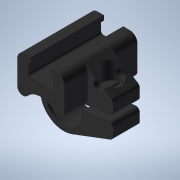
# Autodesk Inventor part: 175091 SMBR-8-8
Saved by Autodesk Inventor 2021 (Build 250183000, 183)
## iProperties
Created: 2026-04-13
Part Number: 175091 SMBR-8-8
Material: Generic
Catalog Web Link: www.3dfindit.com
Description: SMBR-Mounting kit
Vendor: FESTO
Document SubType Name: Modeling
Designer: psAdmin
Manufacturer: FESTO
Mass: 2.14298 g
Surface Area: 20.1199 cm^2
Volume: 2.14298 cm^3
Density: 1 g/cm^3
Appearance: PSOLRGB-176-176-176
Category: PARTsolutions
Company: FESTO
Title: 175091 SMBR-8-8
Author: Cadenas PARTsolutions
Comments: Mounting kit
PSOL_IDENT_0: {$CADENAS_DATA/23d-libs/festo/parts/s/smbr/smbr.prj},169 {VTYP=3D},{NB=175091 SMBR-8-8},{LINA=175091
PSOL_IDENT_1: SMBR-8-8},{NN=SMBR},{DATE=30.08.2023 07:56:14},{GEOMDATE=30.08.2023 07:02:41},{VERSION=},{LINEID=24
PSOL_IDENT_2: 0},{WBVAR=},{WBNUMERIC=}  {NB=175091 SMBR-8-8},{LINA=175091 SMBR-8-8},{KT=DUMMY},{TNR=175091},{TYP=S
PSOL_IDENT_3: MBR-8-8},{INFO=},{B1=18.900},{B2=12.300},{B3=7.000},{B4=0.000},{H1=17.500},{H2=0.000},{H3=0.000},{VE
PSOL_IDENT_4: RS=18.000},{FDTKDM=8},{EOLDATE=},{GTIN=4052568037772}
NB: 175091 SMBR-8-8
NN: SMBR
NT: Mounting kit
NBSYN: $TNR. $TYP.
LINA: 175091 SMBR-8-8
CATALOG: Festo
TNR: 175091
TYP: SMBR-8-8
B1: 18.9
B2: 12.3
B3: 7
B4: 0
H1: 17.5
H2: 0
H3: 0
GTIN: 4052568037772
SUPPLIER: FESTO
ARTICLENO: 175091 SMBR-8-8
BOMINFO: 175091 SMBR-8-8
CREATOR: CADENAS GmbH
Autodesk Inventor part; units mm, degrees
sketch "Skizze_1" plane through (0, 0, 0) normal (0, 0, 1) x (1, 0, 0)
  arc A0 (-6.1, 6.1) -> (2.1523, 0.3923) centre (0, 6.1) ccw
  line L0 (2.1523, 0.3923) -> (12.1528, 4.1634)
  arc A1 (12.1528, 4.1634) -> (12.8, 5.099) centre (11.8, 5.099) ccw
  line L1 (12.8, 5.099) -> (12.8, 7.1459)
  arc A2 (12.8, 7.1459) -> (11.6781, 8.1384) centre (11.8, 7.1459) ccw
  line L2 (11.6781, 8.1384) -> (5.5207, 7.3824)
  arc A3 (5.5207, 7.3824) -> (4.6439, 6.3385) centre (5.6426, 6.3898) ccw
  arc A4 (3.4991, 9.1625) -> (4.6439, 6.3385) centre (0, 6.1) ccw
  arc A5 (3.4991, 9.1625) -> (4.7232, 8.695) centre (4.5526, 10.0845) ccw
  line L3 (4.7232, 8.695) -> (11.9219, 9.5788)
  arc A6 (11.9219, 9.5788) -> (12.8, 10.5714) centre (11.8, 10.5714) ccw
  line L4 (12.8, 10.5714) -> (12.8, 12.6877)
  arc A7 (12.8, 12.6877) -> (12.3421, 13.528) centre (11.8, 12.6877) ccw
  line L5 (12.3421, 13.528) -> (10.513, 14.7078)
  arc A8 (10.513, 14.7078) -> (10.2108, 14.5895) centre (10.4045, 14.5398) ccw
  arc A9 (8.2178, 15.875) -> (10.2108, 14.5895) centre (9, 14.9) ccw
  arc A10 (8.2178, 15.875) -> (8.2011, 16.1991) centre (8.0927, 16.031) ccw
  line L6 (8.2011, 16.1991) -> (5.2841, 18.0807)
  arc A11 (5.2841, 18.0807) -> (4.2, 18.4) centre (4.2, 16.4) ccw
  line L7 (4.2, 18.4) -> (-4.1, 18.4)
  arc A12 (-4.1, 18.4) -> (-6.1, 16.4) centre (-4.1, 16.4) ccw
  line L8 (-6.1, 16.4) -> (-6.1, 6.1)
  constraints: 26 point on circle, 18 end point, 13 centre point
extrude "Extrusion1" add sketch "Skizze_1" along normal mid plane 7
sketch "Skizze_2" plane through (0, 0, 0) normal (0, 0, 1) x (1, 0, 0)
  line L0 (9, 0) -> (9, 18.4)
  line L1 (9, 18.4) -> (11.5, 18.4)
  line L2 (11.5, 18.4) -> (11.5, 11.1)
  line L3 (11.5, 11.1) -> (10.65, 11.1)
  line L4 (10.65, 11.1) -> (10.65, 6.6)
  line L5 (10.65, 6.6) -> (10.25, 6.6)
  line L6 (10.25, 6.6) -> (10.25, 5.1)
  line L7 (10.25, 5.1) -> (10.65, 5.1)
  line L8 (10.65, 5.1) -> (10.65, 0)
  line L9 (10.65, 0) -> (9, 0)
  line L10 (9, 0) -> (9, 18.4)
  constraints: 22 end point
revolve "Revolution1" cut sketch "Skizze_2" angle 360 about axis through (9, 0, 0) along (0, -1, 0)
sketch "Skizze_3" plane through (0, 0, 9.5) normal (0, 0, 1) x (1, 0, 0)
  arc A0 (-6.1, 10.182) -> (-3.478, 9.1864) centre (-4.6, 10.182) ccw
  arc A1 (3.5537, 9.099) -> (-3.478, 9.1864) centre (0, 6.1) ccw
  arc A2 (3.5537, 9.099) -> (6.2, 10.0664) centre (4.7, 10.0664) ccw
  line L0 (6.2, 10.0664) -> (6.2, 16.4)
  arc A3 (6.2, 16.4) -> (4.2, 18.4) centre (4.2, 16.4) ccw
  line L1 (4.2, 18.4) -> (-4.1, 18.4)
  arc A4 (-4.1, 18.4) -> (-6.1, 16.4) centre (-4.1, 16.4) ccw
  line L2 (-6.1, 16.4) -> (-6.1, 10.182)
  constraints: 10 point on circle, 6 end point, 5 centre point
extrude "Extrusion2" add sketch "Skizze_3" against normal blind 6
sketch "Skizze_4" plane through (0, 0, -9.5) normal (0, 0, 1) x (1, 0, 0)
  arc A0 (-6.1, 10.182) -> (-3.478, 9.1864) centre (-4.6, 10.182) ccw
  arc A1 (3.5537, 9.099) -> (-3.478, 9.1864) centre (0, 6.1) ccw
  arc A2 (3.5537, 9.099) -> (6.2, 10.0664) centre (4.7, 10.0664) ccw
  line L0 (6.2, 10.0664) -> (6.2, 16.4)
  arc A3 (6.2, 16.4) -> (4.2, 18.4) centre (4.2, 16.4) ccw
  line L1 (4.2, 18.4) -> (-4.1, 18.4)
  arc A4 (-4.1, 18.4) -> (-6.1, 16.4) centre (-4.1, 16.4) ccw
  line L2 (-6.1, 16.4) -> (-6.1, 10.182)
  constraints: 10 point on circle, 6 end point, 5 centre point
extrude "Extrusion3" add sketch "Skizze_4" along normal blind 6
sketch "Skizze_6" plane through (0, 0, 0) normal (0, 0, 1) x (1, 0, 0)
  line L0 (-3.25, 16.85) -> (-3.25, 14.4)
  arc A0 (-3.25, 14.4) -> (-2.75, 13.9) centre (-2.75, 14.4) ccw
  line L1 (-2.75, 13.9) -> (2.75, 13.9)
  arc A1 (2.75, 13.9) -> (3.25, 14.4) centre (2.75, 14.4) ccw
  line L2 (3.25, 14.4) -> (3.25, 16.85)
  arc A2 (3.25, 16.85) -> (3.05, 17.05) centre (3.05, 16.85) ccw
  line L3 (3.05, 17.05) -> (2.725, 17.05)
  arc A3 (2.525, 17.25) -> (2.725, 17.05) centre (2.725, 17.25) ccw
  line L4 (2.525, 17.25) -> (2.525, 26.3)
  line L5 (2.525, 26.3) -> (-2.525, 26.3)
  line L6 (-2.525, 26.3) -> (-2.525, 17.25)
  arc A4 (-2.725, 17.05) -> (-2.525, 17.25) centre (-2.725, 17.25) ccw
  line L7 (-2.725, 17.05) -> (-3.05, 17.05)
  arc A5 (-3.05, 17.05) -> (-3.25, 16.85) centre (-3.05, 16.85) ccw
  constraints: 16 end point, 12 point on circle, 6 centre point
extrude "Extrusion4" cut sketch "Skizze_6" along normal mid plane 20
sketch "Sketch_1" plane through (0, 0, 0) normal (0, 0, 1) x (1, 0, 0)
  line L0 (9, 3.1) -> (9, 12.7)
  line L1 (9, 12.7) -> (11.1941, 12.7)
  line L2 (11.1941, 12.7) -> (11.25, 11.1)
  line L3 (11.25, 11.1) -> (9.974, 11.1)
  line L4 (9.974, 11.1) -> (10.25, 10.824)
  line L5 (10.25, 10.824) -> (10.25, 3.376)
  line L6 (10.25, 3.376) -> (9.974, 3.1)
  line L7 (9.974, 3.1) -> (9, 3.1)
  line L8 (9, 3.1) -> (9, 12.7)
  constraints: 18 end point
revolve "Revolution2" add sketch "Sketch_1" angle 360 about axis through (9, 3.1, 0) along (0, -1, 0)
thread "Thread1" size "M2.5x0.45" class "6g" standard "ISO Metric profile" full length
sketch "Sketch_2" plane through (9, 12.7, 0) normal (0, 1, 0) x (1, 0, 0)
  line L0 (-0.3, -2.25) -> (0.3, -2.25)
  line L1 (0.3, -2.25) -> (0.3, 2.25)
  line L2 (0.3, 2.25) -> (-0.3, 2.25)
  line L3 (-0.3, 2.25) -> (-0.3, -2.25)
  constraints: 8 end point
extrude "Extrusion5" cut sketch "Sketch_2" against normal blind 0.9
ref_plane "FDT_CYLINDER_XY" through (0, 6.1, 0) normal (0, 0, 1) x (1, 0, 0)
ref_plane "FDT_CYLINDER_YZ" through (0, 6.1, 0) normal (1, 0, 0) x (0, 1, 0)
ref_plane "FDT_CYLINDER_ZX" through (0, 6.1, 0) normal (0, 1, 0) x (0, 0, 1)
ref_plane "FDT_SLOT8_XY" through (0, 13.9, 0) normal (0, 1, 0) x (1, 0, 0)
ref_plane "FDT_SLOT8_YZ" through (0, 13.9, 0) normal (1, 0, 0) x (0, 0, -1)
ref_plane "FDT_SLOT8_ZX" through (0, 13.9, 0) normal (0, 0, -1) x (0, 1, 0)
body "Solid1"
